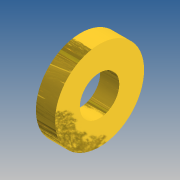
# Autodesk Inventor part: Stepper Motor Rondelle2
Saved by Autodesk Inventor 2012 SP1 (Build 160190100, 190)
## iProperties
Created: 2012-06-26
Part Number: Stepper Motor Rondelle2
Material: Default
Document SubType Name: Modeling
Designer: sta
Density: 1 g/cm^3
Author: sta
Autodesk Inventor part; units mm, degrees
ref_plane "YZ Plane" through (0, 0, 0) normal (1, 0, 0) x (0, 1, 0)
ref_plane "XZ Plane" through (0, 0, 0) normal (0, 1, 0) x (-1, 0, 0)
ref_plane "XY Plane" through (0, 0, 0) normal (0, 0, 1) x (1, 0, 0)
sketch "Sketch1" plane through (0, 0, 0) normal (0, 0, 1) x (1, 0, 0)
  line L0 (0, 0) -> (15.4745, 0) construction
  line L1 (0, 0) -> (0, 3.5)
  line L2 (0, 3.5) -> (1.5, 3.5)
  line L3 (1.5, 3.5) -> (1.5, 0)
  line L4 (0, 1.55) -> (1.5, 1.55)
  line L5 (0, 0) -> (1.5, 0)
  dimension "d0" = 3.1
  dimension "d1" = 7
  dimension "d2" = 1.5
  constraints: 12 end point, 4 perpendicular, 3 point on line, 1 collinear, 1 horizontal
  measures "d0" diameter of L4 L0
  measures "d1" diameter of L2 L0
  measures "d2" distance between parallel lines of L3 L1
revolve "Revolution1" add sketch "Sketch1" angle 360 about axis through (0, 0, 0) along (1, 0, 0) contours L1 L2 L3 L4
body "Solid1"
